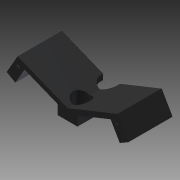
# Autodesk Inventor part: Front Support
Saved by Autodesk Inventor 2015 (Build 190159000, 159)
## iProperties
Created: 2016-02-25
Part Number: Front Support
Material: ABS Plastic
Document SubType Name: Modeling
Designer: James Yelland
Density: 1.06 g/cm^3
Appearance: Smooth - White
Mass: 42.0278 g
Surface Area: 168.788 cm^2
Volume: 39.6489 cm^3
Author: James Yelland
Autodesk Inventor part; units mm, degrees
ref_plane "XZ Plane" through (0, 0, 0) normal (0, 1, 0) x (-1, 0, 0)
ref_plane "XY Plane" through (0, 0, 0) normal (0, 0, 1) x (1, 0, 0)
sketch "Sketch1" plane through (0, 0, 0) normal (0, 1, 0) x (-1, 0, 0)
  line L0 (-56.669873, -1.552559) -> (-61, 0.947441)
  line L1 (56.669873, -1.552559) -> (61, 0.947441)
  line L2 (61, 0.947441) -> (50, 20)
  line L3 (-50, 20) -> (-61, 0.947441)
  line L4 (0, 0) -> (-50, 20)
  line L5 (0, 0) -> (50, 20)
  line L6 (-50, 20) -> (-55, 11.339746)
  line L7 (50, 20) -> (55, 11.339746)
  line L8 (-56.669873, -1.552559) -> (-52.339746, -4.052559)
  line L9 (56.669873, -1.552559) -> (52.339746, -4.052559)
  line L10 (50, 20) -> (52.5, 15.669873)
  line L11 (-50, 20) -> (-52.5, 15.669873)
  line L12 (-43.119361, 11.917617) -> (0, -5.330127)
  line L13 (43.119361, 11.917617) -> (0, -5.330127)
  line L14 (-52.339746, -4.052559) -> (-43.119361, 11.917617)
  line L15 (43.119361, 11.917617) -> (52.339746, -4.052559)
  dimension "d1" = 5
  dimension "d2" = 5
  dimension "d3" = 5
  dimension "d4" = 5
  constraints: 32 end point, 2 midpoint, 2 point on line
  measures "d1" distance of L0.start L8.end
  measures "d2" distance of L1.start L9.end
  measures "d3" distance of L2.end L10.end
  measures "d4" distance of L3.start L11.end
extrude "Extrusion1" add sketch "Sketch1" along normal blind 45
sketch "Sketch2" plane through (0, 0, 0) normal (0, -1, 0) x (1, 0, 0)
  line L0 (61, 0.947441) -> (52.339746, -4.052559)
  line L1 (50, 20) -> (61, 0.947441)
  line L2 (0, 0) -> (50, 20)
  line L3 (-50, 20) -> (0, 0)
  line L4 (-61, 0.947441) -> (-50, 20)
  line L5 (-52.339746, -4.052559) -> (-61, 0.947441)
  line L6 (-43.119361, 11.917617) -> (-52.339746, -4.052559)
  line L7 (0, -5.330127) -> (-43.119361, 11.917617)
  line L8 (43.119361, 11.917617) -> (0, -5.330127)
  line L9 (52.339746, -4.052559) -> (43.119361, 11.917617)
  line L10 (-56.669873, -1.552559) -> (-49.169873, 11.437822)
  line L11 (56.669873, -1.552559) -> (49.169873, 11.437822)
  circle A0 centre (49.169873, 11.437822) radius 1.4
  circle A1 centre (-49.169873, 11.437822) radius 1.4
  dimension "d8" = 15
  dimension "d9" = 15
  dimension "d10" = 2.8
  dimension "d11" = 2.8
  constraints: 4 end point, 2 centre point, 2 coincident, 2 midpoint
  measures "d8" distance of L10.start L10.end
  measures "d9" distance of L11.start L11.end
  measures "d10" diameter of A0
  measures "d11" diameter of A1
extrude "Extrusion2" cut sketch "Sketch2" against normal blind 30 contours A0 | A1
sketch "Sketch3" plane through (0, 45, 0) normal (0, 1, 0) x (1, 0, 0)
  circle A0 centre (-54.169873, -2.777568) radius 1.4
  circle A1 centre (54.169873, -2.777568) radius 1.4
  line L0 (61, -0.947441) -> (52.339746, 4.052559)
  line L1 (52.339746, 4.052559) -> (43.119361, -11.917617)
  line L2 (43.119361, -11.917617) -> (0, 5.330127)
  line L3 (0, 5.330127) -> (-43.119361, -11.917617)
  line L4 (-43.119361, -11.917617) -> (-52.339746, 4.052559)
  line L5 (-52.339746, 4.052559) -> (-61, -0.947441)
  line L6 (-61, -0.947441) -> (-50, -20)
  line L7 (-50, -20) -> (0, 0)
  line L8 (0, 0) -> (50, -20)
  line L9 (50, -20) -> (61, -0.947441)
  dimension "d30" = 2.8
  dimension "d31" = 2.8
  constraints: 2 centre point
  measures "d30" diameter of A0
  measures "d31" diameter of A1
extrude "Extrusion3" cut sketch "Sketch3" against normal blind 20 contours A0 | A1
chamfer "Chamfer1" distance 1 angle 45 2 edges at (-56.6699, 45, -1.5526) (56.6699, 45, -1.5526)
chamfer "Chamfer2" distance 1 angle 45 8 edges at (55.25, 45, 10.9067) (47.4796, 45, 4.3655) (21.5597, 45, 3.2937) (-21.5597, 45, 3.2937) (-47.4796, 45, 4.3655) (-55.25, 45, 10.9067) (-25, 45, 10) (25, 45, 10)
ref_plane "Work Plane1" through (0, 0, 0) normal (0, 0, -1) x (0, 1, 0)
sketch "Sketch4" plane through (0, 0, 0) normal (0, 0, -1) x (0, 1, 0)
  line L0 (0, 0) -> (0, -10)
  line L1 (0, 0) -> (0, -43.119361)
  line L2 (0, -10) -> (25, -10)
  line L3 (25, -10) -> (25, 10)
  line L4 (25, 10) -> (0, 10)
  line L5 (0, 10) -> (0, 0)
  dimension "d33" = 10
  dimension "d34" = 25
  dimension "d35" = 20
  constraints: 10 end point, 3 perpendicular, 1 collinear, 1 point on line
  measures "d33" distance of L0.start L0.end
  measures "d34" distance of L0.end L2.end
  measures "d35" distance of L2.end L3.end
extrude "Extrusion4" add sketch "Sketch4" along normal blind 11
sketch "Sketch5" plane through (0, 0, -11) normal (0, 0, -1) x (-1, 0, 0)
  circle A0 centre (0, 14) radius 8.5
  circle A1 centre (-7.5, 7.5) radius 0.9
  circle A2 centre (7.5, 7.5) radius 0.9
  line L0 (0, 14) -> (0, 41)
  line L1 (0, 0) -> (0, 44)
  line L2 (-8.5, 41) -> (-8.5, 45)
  line L3 (0, 45) -> (-43.552262, 45)
  line L4 (8.5, 41) -> (8.5, 45)
  line L5 (0, 45) -> (49.567099, 45)
  line L6 (8.5, 45) -> (-8.5, 45)
  arc A3 (-8.5, 41) -> (8.5, 41) centre (0, 41) ccw
  dimension "d38" = 17
  dimension "d39" = 1.8
  dimension "d40" = 1.8
  dimension "d41" = 27
  constraints: 8 end point, 4 centre point, 3 point on line, 2 point on circle, 1 horizontal, 1 parallel, 1 vertical
  measures "d38" diameter of A0
  measures "d39" diameter of A1
  measures "d40" diameter of A2
  measures "d41" distance of L0.start L0.end
extrude "Extrusion5" cut sketch "Sketch5" against normal through all contours A0 L1 L0 | L0 L1 A0 | L2 L3 L5 L4 A3
chamfer "Chamfer3" distance 1 angle 45 2 edges at (8.5, 45, 0.7349) (-8.5, 45, 0.7349)
sketch "Sketch6" plane through (0, 0, -11) normal (0, 0, -1) x (-1, 0, 0)
  circle A0 centre (-7.5, 7.5) radius 0.9
  circle A1 centre (7.5, 7.5) radius 0.9
  point P0 (0, 0)
  point P1 (0, 0)
  dimension "d49" = 1.8
  dimension "d50" = 1.8
  constraints: 2 centre point
  measures "d49" diameter of A0
  measures "d50" diameter of A1
extrude "Extrusion6" cut sketch "Sketch6" against normal blind 10
sketch "Sketch7" plane through (0, 0, -11) normal (0, 0, -1) x (-1, 0, 0)
  line L0 (-10, 25) -> (10, 25)
  line L1 (-10, 25) -> (-6, 25)
  line L2 (-6, 25) -> (-6, 21)
  line L3 (-6, 21) -> (-10, 21)
  line L4 (10, 25) -> (6, 25)
  line L5 (-10, 25) -> (10, 25)
  line L6 (6, 25) -> (6, 21)
  line L7 (6, 21) -> (10, 21)
  line L8 (10, 25) -> (10, 21)
  line L9 (-10, 25) -> (-6, 25)
  line L10 (-6, 25) -> (-6, 21)
  line L11 (-6, 21) -> (-10, 21)
  line L12 (-10, 21) -> (-10, 25)
  line L13 (6, 25) -> (10, 25)
  line L14 (10, 25) -> (10, 21)
  line L15 (10, 21) -> (6, 21)
  line L16 (6, 21) -> (6, 25)
  dimension "d54" = 4
  dimension "d55" = 4
  dimension "d56" = 4
  constraints: 34 end point, 5 perpendicular, 4 parallel, 2 horizontal, 1 point on line
  measures "d54" distance of L2.start L2.end
  measures "d55" distance of L8.start L16.end
  measures "d56" distance of L16.end L7.start
extrude "Extrusion7" cut sketch "Sketch7" against normal blind 4
fillet "Fillet1" radius 1 2 edges at (6, 21, -9) (-6, 21, -9)
body "Solid1"
